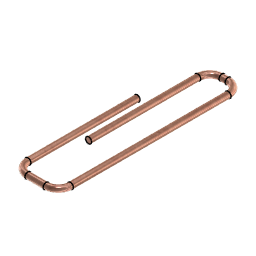
Paper-Clip-1 (Autodesk Fusion 360 design; units mm, degrees)
Autodesk Fusion 360 part; units mm, degrees
sketch "Sketch1" plane through (0, 0, 0) normal (0, 0, 1) x (1, 0, 0)
  line L0 (0, 0) -> (0, 90)
  line L1 (10, 100) -> (15, 100)
  line L2 (25, 90) -> (25, -40)
  line L3 (15, -50) -> (0, -50)
  line L4 (-10, -40) -> (-10, 50)
  arc A0 (25, 90) -> (15, 100) centre (15, 90) ccw
  arc A1 (10, 100) -> (0, 90) centre (10, 90) ccw
  arc A2 (15, -50) -> (25, -40) centre (15, -40) ccw
  arc A3 (-10, -40) -> (0, -50) centre (0, -40) ccw
  point P0 (0, 100)
  point P1 (25, 100)
  point P2 (25, -50)
  point P3 (-10, -50)
  dimension "d3" = 100
  dimension "d4" = 25
  dimension "d5" = 150
  dimension "d6" = 35
  dimension "d7" = 100
  dimension "d8" = 10
  dimension "d9" = 10
  dimension "d10" = 10
  dimension "d11" = 10
  constraint coincident L0.start origin
  constraint vertical L0
  constraint perpendicular L0 L1
  constraint perpendicular L1 L2
  constraint perpendicular L2 L3
  constraint perpendicular L3 L4
  constraint coincident P1 L1
  constraint coincident P1 L2
  constraint tangent L1 A0
  constraint tangent L2 A0
  constraint coincident P0 L0
  constraint coincident P0 L1
  constraint tangent L0 A1
  constraint tangent L1 A1
  constraint coincident P2 L2
  constraint coincident P2 L3
  constraint tangent L2 A2
  constraint tangent L3 A2
  constraint coincident P3 L3
  constraint coincident P3 L4
  constraint tangent L3 A3
  constraint tangent L4 A3
  measures "d3" distance of L0.start P0
  measures "d4" distance of P0 P1
  measures "d5" distance of P1 P2
  measures "d6" distance of P2 P3
  measures "d7" distance of P3 L4.end
  measures "d8" radius of A0
  measures "d9" radius of A1
  measures "d10" radius of A2
  measures "d11" radius of A3
pipe "Pipe1" add diameter 5 path "Sketch1" along L4 A3 L3 A2 L2 A0 L1 A1 L0
sketch "Sketch2" plane through (0, 0, 0) normal (0, 0, 1) x (1, 0, 0)
